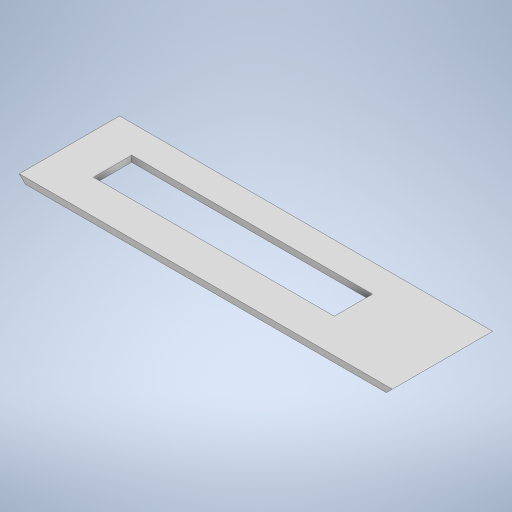
# Autodesk Inventor part: Front Wall
Saved by Autodesk Inventor 2023 (Build 270158000, 158)
## iProperties
Created: 2023-02-06
Part Number: Front Wall
Material: Generic
Document SubType Name: Modeling
Designer: Ahmed Nazir
Density: 1 g/cm^3
Appearance: Default
Author: Ahmed Nazir
Autodesk Inventor part; units mm, degrees
ref_plane "YZ Plane" through (0, 0, 0) normal (1, 0, 0) x (0, 1, 0)
ref_plane "XZ Plane" through (0, 0, 0) normal (0, 1, 0) x (-1, 0, 0)
ref_plane "XY Plane" through (0, 0, 0) normal (0, 0, 1) x (1, 0, 0)
sketch "Sketch1" plane through (0, 0, 0) normal (0, 1, 0) x (-1, 0, 0)
  line L0 (93, -25) -> (-93, -25)
  line L1 (-93, -25) -> (-93, 25)
  line L2 (-93, 25) -> (93, 25)
  line L3 (93, 25) -> (93, -25)
  line L4 (93, -25) -> (-93, 25) construction
  line L5 (-93, -25) -> (93, 25) construction
  line L6 (73, -11) -> (-47, -11)
  line L7 (-47, -11) -> (-47, 8)
  line L8 (-47, 8) -> (73, 8)
  line L9 (73, 8) -> (73, -11)
  point P0 (0, 0)
  dimension "d0" = 186
  dimension "d1" = 50
  dimension "d2" = 17
  dimension "d3" = 36
  dimension "d4" = 120
  dimension "d5" = 20
  constraints: 20 end point, 4 parallel, 2 horizontal, 2 midpoint, 2 perpendicular
  measures "d0" distance of L1.end L2.end
  measures "d1" distance of L0.end L1.end
  measures "d2" distance between parallel lines of L2 L8
  measures "d3" distance between parallel lines of L2 L6
  measures "d4" distance of L6.start L6.end
  measures "d5" distance between parallel lines of L3 L9
extrude "Extrusion1" add sketch "Sketch1" along normal blind 3
chamfer "Chamfer3" distance 3 angle 45 1 edges at (-93, 0, 0) measured on face at (-93, 1, -8.3333)
chamfer "Chamfer4" distance 3 angle 45 1 edges at (93, 0, 0) measured on face at (93, 1, 8.3333)
body "Solid1"
